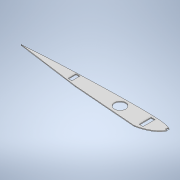
# Autodesk Inventor part: airfoil
Saved by Autodesk Inventor 2021 (Build 250183000, 183)
## iProperties
Created: 2021-03-06
Part Number: airfoil
Material: Generic
Document SubType Name: Modeling
Designer: Ferdinand Hubbard
Density: 1 g/cm^3
Appearance: Default
Author: Ferdinand Hubbard
Autodesk Inventor part; units mm, degrees
ref_plane "YZ Plane" through (0, 0, 0) normal (1, 0, 0) x (0, 1, 0)
ref_plane "XZ Plane" through (0, 0, 0) normal (0, 1, 0) x (-1, 0, 0)
ref_plane "XY Plane" through (0, 0, 0) normal (0, 0, 1) x (1, 0, 0)
sketch "Sketch1" plane through (0, 0, 0) normal (0, 1, 0) x (-1, 0, 0)
  spline S0 degree 5 poles (51.979, 34.2431) (50.8625, 34.028) (47.6122, 33.3669) (42.4356, 32.1484) (35.6445, 30.1748) (27.6551, 26.8948) (19.9185, 23.282) (13.2966, 18.4115) (8.2164, 15.1418) (4.1239, 9.095) (1.8688, 7.6936) (0.0614, 1.3934) (-0.0327, 0.731) (0.0012, -0.8157) (0.1601, -1.4322) (0.3844, -2.0614) (0.8781, -2.5552) (1.4257, -3.0265) (3.0955, -4.0074) (3.6639, -4.2019) (12.8054, -7.5819) (15.4761, -7.0321) (27.2625, -9.6881) (35.794, -9.6188) (49.4051, -10.751) (62.7459, -10.7975) (78.537, -11.1277) (95.0547, -11.0417) (112.8972, -10.9363) (131.4585, -10.6401) (150.706, -10.2647) (170.3212, -9.7779) (190.1154, -9.2196) (209.8264, -8.5865) (229.2522, -7.9015) (248.1108, -7.1621) (266.2978, -6.3832) (283.3653, -5.5497) (299.6157, -4.6319) (313.9444, -3.6518) (328.0305, -2.6976) (338.3237, -1.8152) (350.4289, -1.1113) (355.0714, -0.5725) (365.0696, -0.2501) (365.4645, -0.0704) (369.2011, -0.021) (369.9991, -0.0065) (370, 0) (370.0001, 0.0004) (369.9988, 0.0007) (369.9962, 0.0011) (369.9924, 0.0014) (369.9872, 0.0018) knots 0.394181 0.394181 0.394181 0.394181 0.394181 0.394181 0.402168 0.417605 0.432338 0.446343 0.459583 0.472 0.483512 0.493356 0.501621 0.508282 0.513504 0.517523 0.521304 0.525161 0.529372 0.535087 0.54267 0.552364 0.564195 0.578324 0.593841 0.610553 0.628313 0.64698 0.666409 0.686456 0.706982 0.727856 0.748948 0.770129 0.791274 0.812253 0.83294 0.853208 0.872937 0.892004 0.91028 0.927618 0.943841 0.958715 0.971915 0.982888 0.99083 1 1 1 1 1 1.000508 1.000508 1.000508 1.000508 1.000508 1.000508
  circle A0 centre (370, 0) radius 160 construction
  line L0 (370, 0) -> (211.4974, 21.8387)
  circle A1 centre (211.4974, 21.8387) radius 160 construction
  line L1 (211.4974, 21.8387) -> (51.979, 34.2431)
  circle A2 centre (112.1091, 9.1521) radius 14.25
  circle A3 centre (112.1091, 9.1521) radius 9.25 construction
  line L2 (38.0597, 25.4533) -> (48.0597, 25.4533)
  line L3 (48.0597, 25.4533) -> (48.0597, -4.5467)
  line L4 (48.0597, -4.5467) -> (38.0597, -4.5467)
  line L5 (38.0597, -4.5467) -> (38.0597, 25.4533)
  line L6 (227.007, 15.0223) -> (237.007, 15.0223)
  line L7 (237.007, 15.0223) -> (237.007, -4.9777)
  line L8 (237.007, -4.9777) -> (227.007, -4.9777)
  line L9 (227.007, -4.9777) -> (227.007, 15.0223)
  line L10 (-0.096, 2.719) -> (4.904, 2.719)
  line L11 (4.904, 2.719) -> (4.904, -2.281)
  line L12 (4.904, -2.281) -> (-0.096, -2.281)
  line L13 (-0.096, -2.281) -> (-0.096, 2.719)
  point P0 (0, 0)
  point P1 (35.937, 30.0257)
  point P2 (27.0238, 26.4761)
  point P3 (19.2974, 22.4624)
  point P4 (12.8156, 18.139)
  point P5 (7.6237, 13.6489)
  point P6 (3.7499, 9.1521)
  point P7 (1.2115, 4.8535)
  point P8 (0.0668, 1.0195)
  point P9 (0.0003, -0.0638)
  point P10 (0.0755, -0.9849)
  point P11 (0.2106, -1.5356)
  point P12 (0.4302, -2.0122)
  point P13 (0.7739, -2.4345)
  point P14 (1.2488, -2.8423)
  point P15 (2.1566, -3.4383)
  point P16 (3.2773, -4.0196)
  point P17 (8.2772, -5.8071)
  point P18 (15.3669, -7.4261)
  point P19 (24.3167, -8.7706)
  point P20 (35.0526, -9.7678)
  point P21 (47.5438, -10.4262)
  point P22 (61.6814, -10.8267)
  point P23 (77.2847, -11.0213)
  point P24 (94.162, -11.0379)
  point P25 (112.1091, -10.9014)
  point P26 (130.911, -10.6315)
  point P27 (150.3435, -10.2474)
  point P28 (170.176, -9.7646)
  point P29 (190.1737, -9.1986)
  point P30 (210.0997, -8.5616)
  point P31 (229.7182, -7.8653)
  point P32 (248.7963, -7.1166)
  point P33 (267.1071, -6.3194)
  point P34 (284.4371, -5.4606)
  point P35 (300.619, -4.5258)
  point P36 (315.5184, -3.5432)
  point P37 (328.988, -2.5786)
  point P38 (340.8625, -1.7041)
  point P39 (350.9622, -0.9861)
  point P40 (359.0984, -0.4682)
  point P41 (365.0855, -0.1602)
  point P42 (368.7597, -0.0285)
  point P43 (369.9872, 0.0018)
  point P44 (0.4871, 2.719)
  point P45 (0.63, -2.281)
  dimension "d5" = 160
  dimension "d8" = 160
  dimension "d9" = 28.5
  dimension "d10" = 18.5
  dimension "d11" = 10
  dimension "d12" = 30
  dimension "d13" = 10
  dimension "d14" = 20
  dimension "d17" = 5
  dimension "d18" = 5
  constraints: 28 end point, 6 parallel, 3 horizontal, 3 perpendicular, 2 centre point, 1 coincident, 1 point on line, 53 other
  measures "d5" distance of L0.end L0.start
  measures "d8" distance of L0.end L1.end
  measures "d9" diameter of A2
  measures "d10" diameter of A3
  measures "d11" distance of L3.end L4.end
  measures "d12" distance of L2.end L3.end
  measures "d13" distance of L7.end L8.end
  measures "d14" distance of L6.end L7.end
  measures "d17" distance of L11.end L12.end
  measures "d18" distance of L10.end L11.end
extrude "Extrusion2" add sketch "Sketch1" along normal blind 2 contours S0 L12 L11 L10 L1 L0
body "Solid2"
